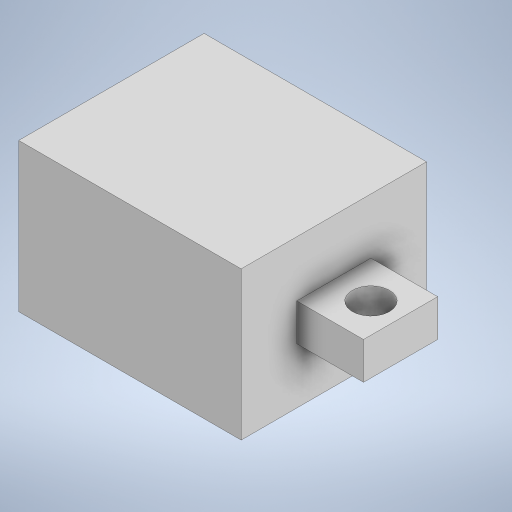
# Autodesk Inventor part: head
Saved by Autodesk Inventor 2024 (Build 280153000, 153)
## iProperties
Created: 2023-10-16
Part Number: head
Material: Generic
Document SubType Name: Modeling
Designer: Piter
Density: 1 g/cm^3
Appearance: Default
Author: Piter
Autodesk Inventor part; units mm, degrees
ref_plane "YZ Plane" through (0, 0, 0) normal (1, 0, 0) x (0, 1, 0)
ref_plane "XZ Plane" through (0, 0, 0) normal (0, 1, 0) x (-1, 0, 0)
ref_plane "XY Plane" through (0, 0, 0) normal (0, 0, 1) x (1, 0, 0)
sketch "Sketch1" plane through (0, 0, 0) normal (0, 1, 0) x (-1, 0, 0)
  line L0 (0, 0) -> (30, 0)
  line L1 (30, 0) -> (30, -25)
  line L2 (30, -25) -> (0, -25)
  line L3 (0, -25) -> (0, 0)
  dimension "d0" = 30
  dimension "d1" = 25
  constraints: 8 end point, 2 parallel, 1 horizontal, 1 perpendicular
  measures "d0" distance of L1.end L2.end
  measures "d1" distance of L0.end L1.end
extrude "Extrusion1" add sketch "Sketch1" along normal blind 20
sketch "Sketch2" plane through (0, 0, 0) normal (0, -1, 0) x (1, 0, 0)
  circle A0 centre (-20, -12.5) radius 2.5
  line L0 (0, 0) -> (0, -25) projected
  point P0 (0, -12.5)
  dimension "d4" = 5
  dimension "d15" = 20
  constraints: 1 centre point, 1 midpoint
  measures "d4" diameter of A0
  measures "d15" distance of point (0, -12.5) A0.centre
extrude "Extrusion2" cut sketch "Sketch2" against normal blind 5
sketch "Sketch3" plane through (0, 0, 0) normal (1, 0, 0) x (0, 0, -1)
  line L0 (17.5, 7.5) -> (7.5, 7.5)
  line L1 (7.5, 7.5) -> (7.5, 12.5)
  line L2 (7.5, 12.5) -> (17.5, 12.5)
  line L3 (17.5, 12.5) -> (17.5, 7.5)
  line L4 (17.5, 7.5) -> (7.5, 12.5) construction
  line L5 (7.5, 7.5) -> (17.5, 12.5) construction
  point P0 (0, 0)
  point P1 (12.5, 10)
  dimension "d7" = 10
  dimension "d8" = 5
  constraints: 12 end point, 2 midpoint, 2 parallel, 1 horizontal, 1 perpendicular
  measures "d7" distance of L1.end L2.end
  measures "d8" distance of L0.end L1.end
extrude "Extrusion3" add sketch "Sketch3" along normal blind 9
sketch "Sketch4" plane through (0, 12.5, -7.5) normal (0, 1, 0) x (1, 0, 0)
  circle A0 centre (5, 5) radius 2.5
  line L0 (0, -7.5) -> (0, 17.5) projected
  dimension "d11" = 5
  dimension "d14" = 5
  constraints: 1 centre point
  measures "d11" diameter of A0
  measures "d14" distance from line of A0.centre L0
extrude "Extrusion4" cut sketch "Sketch4" against normal through all
body "Solid1"
